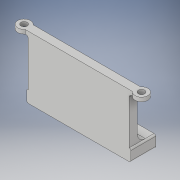
# Autodesk Inventor part: License_plate_mount
Saved by Autodesk Inventor 2019 (Build 230136000, 136)
## iProperties
Created: 2019-09-02
Part Number: License_plate_mount
Material: Generic
Document SubType Name: Modeling
Designer: steve
Density: 1 g/cm^3
Appearance: Default
Author: steve
Autodesk Inventor part; units mm, degrees
ref_plane "YZ Plane" through (0, 0, 0) normal (1, 0, 0) x (0, 1, 0)
ref_plane "XZ Plane" through (0, 0, 0) normal (0, 1, 0) x (-1, 0, 0)
ref_plane "XY Plane" through (0, 0, 0) normal (0, 0, 1) x (1, 0, 0)
sketch "Sketch1" plane through (0, 0, 0) normal (0, 0, 1) x (1, 0, 0)
  line L0 (2, 0) -> (128, 0)
  line L1 (130, 2) -> (130, 13)
  line L2 (128, 15) -> (2, 15)
  line L3 (0, 13) -> (0, 2)
  arc A0 (130, 13) -> (128, 15) centre (128, 13) ccw
  arc A1 (128, 0) -> (130, 2) centre (128, 2) ccw
  arc A2 (0, 2) -> (2, 0) centre (2, 2) ccw
  arc A3 (2, 15) -> (0, 13) centre (2, 13) ccw
  point P0 (0, 0)
  point P1 (130, 15)
  point P2 (130, 0)
  point P3 (0, 15)
  dimension "d0" = 130
  dimension "d1" = 15
  dimension "d2" = 2
  constraints: 8 end point, 8 point on circle, 8 point on line, 8 tangent, 4 centre point, 3 equal radius, 2 parallel, 1 horizontal, 1 perpendicular
  measures "d0" distance of point (130, 15) point (0, 15)
  measures "d1" distance of point (130, 0) point (130, 15)
  measures "d2" radius of A0
extrude "Extrusion1" add sketch "Sketch1" along normal blind 31
sketch "Sketch2" plane through (2, 15, 0) normal (0, 1, 0) x (1, 0, 0)
  line L0 (126, -21) -> (0, -21)
  line L1 (0, -21) -> (0, -31)
  line L2 (0, -31) -> (126, -31)
  line L3 (126, -31) -> (126, -21)
  line L4 (126, 0) -> (126, -31) projected
  line L5 (0, 0) -> (0, -31) projected
  line L6 (126, -31) -> (0, -31) projected
  point P0 (-2, 0)
  dimension "d5" = 10
  constraints: 8 end point, 3 collinear, 2 parallel, 1 horizontal, 1 perpendicular
  measures "d5" distance between parallel lines of L2 L0
extrude "Extrusion2" add sketch "Sketch2" along normal blind 58
fillet "Fillet1" radius 10 1 edges at (65, 15, 21)
sketch "Sketch3" plane through (2, 73, 0) normal (0, 1, 0) x (1, 0, 0)
  arc A0 (130.005, -31) -> (130.005, -21) centre (136.25, -26) ccw
  arc A1 (-4.005, -21) -> (-4.005, -31) centre (-10.25, -26) ccw
  line L0 (0, -31) -> (126, -31) projected
  line L1 (63, 10.8674) -> (63, -51.873)
  line L2 (126, -21) -> (0, -21) projected
  line L3 (126, -21) -> (0, -21)
  line L4 (0, -31) -> (126, -31)
  line L5 (-2, -31) -> (0, -31) projected
  line L6 (0, -31) -> (-4.005, -31)
  line L7 (0, -21) -> (-4.005, -21)
  line L8 (126, -21) -> (130.005, -21)
  line L9 (126, -31) -> (130.005, -31)
  circle A2 centre (-10.25, -26) radius 4
  circle A3 centre (136.25, -26) radius 4
  point P0 (-2, 0)
  dimension "d11" = 16
  dimension "d13" = 126
  dimension "d14" = 146.5
  dimension "d16" = 73.25
  dimension "d17" = 63
  dimension "d18" = 10
  dimension "d19" = 5
  dimension "d20" = 5
  dimension "d27" = 8
  constraints: 14 end point, 4 centre point, 4 point on circle, 3 collinear, 2 coincident, 2 equal radius, 2 point on line, 1 parallel, 1 vertical
  measures "d11" diameter of A0
  measures "d13" distance of L0.start L0.end
  measures "d14" distance of A1.centre A0.centre
  measures "d16" distance from line of A0.centre L1
  measures "d17" distance from line of L0.start L1
  measures "d18" distance between parallel lines of L2 L0
  measures "d19" distance from line of L0 A0.centre
  measures "d20" distance from line of L0 A1.centre
  measures "d27" diameter of A3
extrude "Extrusion4" add sketch "Sketch3" along normal blind 5
fillet "Fillet4" radius 3 2 edges at (2, 73, 26) (128, 73, 26)
equation "\"d16\" = 0.5 * d14"
equation "\"d17\" = 0.5 * d13"
equation "\"d19\" = 0.5 * d18"
equation "\"d20\" = d19"
body "Solid1"
